PasseCable (Autodesk Fusion 360 design; units mm, degrees)
Autodesk Fusion 360 part; units mm, degrees
sketch "Sketch2" plane through (0, 0, 0) normal (0, 1, 0) x (1, 0, 0)
  line L0 (7.5, 10) -> (-7.5, 10)
  line L1 (-7.5, 10) -> (-7.5, -10)
  line L2 (-7.5, -10) -> (7.5, -10)
  line L3 (7.5, -10) -> (7.5, 10)
  line L4 (7.5, 10) -> (-7.5, -10) construction
  line L5 (-7.5, 10) -> (7.5, -10) construction
  line L6 (-7.5, 0) -> (7.5, 0) construction
  line L7 (-7.5, 3) -> (-5, 3)
  line L8 (-5, 3) -> (-5, -3)
  line L9 (-5, -3) -> (-7.5, -3)
  line L10 (-7.5, -3) -> (-7.5, 3)
  line L11 (-7.5, 3) -> (-5, -3) construction
  line L12 (-5, 3) -> (-7.5, -3) construction
  line L13 (7.5, 3) -> (5, 3)
  line L14 (5, 3) -> (5, -3)
  line L15 (5, -3) -> (7.5, -3)
  line L16 (7.5, -3) -> (7.5, 3)
  line L17 (7.5, 3) -> (5, -3) construction
  line L18 (5, 3) -> (7.5, -3) construction
  circle A0 centre (0, 0) radius 2.1
  point P0 (-6.25, 0)
  point P1 (6.25, 0)
  dimension "d1" = 15
  dimension "d2" = 20
  dimension "d3" = 2.5
  dimension "d4" = 6
  dimension "d5" = 6
  dimension "d6" = 2.5
  dimension "d7" = 4.2
  constraint horizontal L0
  constraint perpendicular L0 L1
  constraint parallel L0 L2
  constraint parallel L1 L3
  constraint coincident L4 A0.centre
  constraint coincident L5 A0.centre
  constraint coincident A0.centre origin
  constraint midpoint L1 L6.start
  constraint midpoint L3 L6.end
  constraint horizontal L7
  constraint perpendicular L7 L8
  constraint parallel L7 L9
  constraint parallel L8 L10
  constraint coincident L11 P0
  constraint coincident L12 P0
  constraint coincident L6 P0
  constraint coincident L1 L7.start
  constraint horizontal L13
  constraint perpendicular L13 L14
  constraint parallel L13 L15
  constraint parallel L14 L16
  constraint coincident L3 L13.start
  constraint coincident L17 P1
  constraint coincident L18 P1
  constraint coincident L6 P1
  measures "d1" distance of L1.end L2.end
  measures "d2" distance of L0.end L1.end
  measures "d3" distance of L8.end L9.end
  measures "d4" distance of L7.end L8.end
  measures "d5" distance of L13.end L14.end
  measures "d6" distance of L14.end L15.end
  measures "d7" diameter of A0
extrude "Extrude1" add sketch "Sketch2" against normal blind 2 contours L3 L13 L14 L15 L16 | L1 L7 L8 L9 L10 makes body 1 at (-6.6667, 0, -1) makes body 2 at (5.8333, 0, 1)
extrude "Extrude2" add sketch "Sketch2" along normal blind 5 bodies 1 2
chamfer "Chamfer1" distance 2 angle 45 2 edges at (-6.25, -2, -3) (6.25, -2, -3) on bodies 1
sketch "Sketch3" plane through (0, 5, 0) normal (0, 1, 0) x (-1, 0, 0)
  circle A0 centre (0, 0) radius 2.1
  line L0 (7.5, -10) -> (7.5, 10)
  line L1 (7.5, 10) -> (-7.5, 10)
  line L2 (-7.5, 10) -> (-7.5, -10)
  line L3 (-7.5, -10) -> (7.5, -10)
  circle A1 centre (0, 0) radius 5
  line L4 (-7.5, 10) -> (-5.5, 10)
  line L5 (-5.5, 10) -> (-5.5, -10)
  line L6 (-5.5, -10) -> (-7.5, -10)
  line L7 (-7.5, -10) -> (-7.5, 10)
  line L8 (7.5, 10) -> (5.5, 10)
  line L9 (5.5, 10) -> (5.5, -10)
  line L10 (5.5, -10) -> (7.5, -10)
  line L11 (7.5, -10) -> (7.5, 10)
  dimension "d13" = 10
  dimension "d16" = 2
  dimension "d17" = 2
  constraint coincident A0.centre A1.centre
  constraint horizontal L4
  constraint vertical L5
  constraint horizontal L6
  constraint vertical L7
  constraint coincident L3 L5.end
  constraint coincident L1.end L2.start
  constraint horizontal L8
  constraint vertical L9
  constraint horizontal L10
  constraint vertical L11
  constraint coincident L3 L9.end
  constraint coincident L0.end L1.start
  measures "d13" diameter of A1
  measures "d16" distance of L1.end L4.end
  measures "d17" distance of L0.end L8.end
extrude "Extrude3" cut sketch "Sketch3" against normal blind 3 contours A1 bodies 1
extrude "Extrude4" add sketch "Sketch3" along normal blind 5 contours L0 L1 L3 L8 L9 L10 L11 | L1 L2 L3 L4 L5 L6 L7 bodies 1
fillet "Fillet1" radius 5 1 edges at (0, 5, 10) on bodies 1
fillet "Fillet2" radius 4.5 4 edges at (5.5, 3.5355, 8.5355) (5.5, 5, -2.5) (-5.5, 5, -2.5) (-5.5, 3.5355, 8.5355) on bodies 1
fillet "Fillet3" radius 1 4 edges at (7.5, 10, 0) (5.5, 10, 0) (-5.5, 10, 0) (-7.5, 10, 0) on bodies 1
sketch "Sketch4" plane through (7.5, 0, 0) normal (1, 0, 0) x (0, 1, 0)
  line L0 (9, -10) -> (9, 10)
  line L1 (9, 10) -> (0, 10)
  line L2 (0, 10) -> (0, 3)
  line L3 (0, 3) -> (-2, 3)
  line L4 (-2, 3) -> (-2, -1)
  line L5 (-2, -1) -> (0, -3)
  line L6 (0, -3) -> (0, -10)
  line L7 (0, -10) -> (9, -10)
  line L8 (0, 0) -> (9, 0) construction
  line L9 (5, 10) -> (5, -10) construction
  line L10 (5, 8) -> (7, 8)
  line L11 (7, 8) -> (7, 3)
  line L12 (7, 3) -> (5, 3)
  line L13 (5, 3) -> (5, 8)
  line L14 (5, -8) -> (7, -8)
  line L15 (7, -8) -> (7, -3)
  line L16 (7, -3) -> (5, -3)
  line L17 (5, -3) -> (5, -8)
  dimension "d24" = 5
  dimension "d25" = 2
  dimension "d26" = 5
  dimension "d27" = 2
  constraint coincident L8.start origin
  constraint midpoint L0 L8.end
  constraint coincident L1 L9.start
  constraint coincident L7 L9.end
  constraint perpendicular L7 L9
  constraint horizontal L10
  constraint vertical L11
  constraint horizontal L12
  constraint vertical L13
  constraint coincident L9 L10.start
  constraint symmetric L8 L10.start L14.start
  constraint symmetric L8 L10.end L14.end
  constraint symmetric L8 L11.end L15.end
  constraint symmetric L8 L12.end L16.end
  measures "d24" distance of L8.start L9
  measures "d25" distance of L10.start L10.end
  measures "d26" distance of L10.start L12.end
  measures "d27" distance of L9.start L10.start
extrude "Extrude5" cut sketch "Sketch4" against normal through all contours L10 L11 L12 L13 | L14 L15 L16 L17 bodies 1
